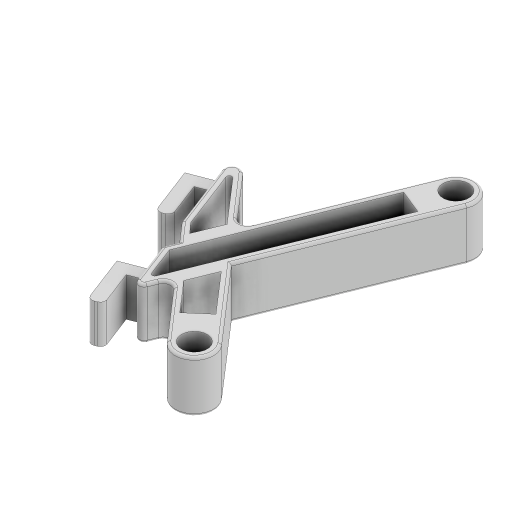
# Autodesk Inventor part: biellaa
Saved by Autodesk Inventor 2024 (Build 280153000, 153)
## iProperties
Created: 2024-04-18
Part Number: biellaa
Material: Generic
Document SubType Name: Modeling
Designer: alexz
Density: 1 g/cm^3
Appearance: Default
Author: alexz
Autodesk Inventor part; units mm, degrees
ref_plane "YZ Plane" through (0, 0, 0) normal (1, 0, 0) x (0, 1, 0)
ref_plane "XZ Plane" through (0, 0, 0) normal (0, 1, 0) x (-1, 0, 0)
ref_plane "XY Plane" through (0, 0, 0) normal (0, 0, 1) x (1, 0, 0)
sketch "Sketch1" plane through (0, 0, 0) normal (0, 1, 0) x (-1, 0, 0)
  circle A0 centre (0, 0) radius 5
  circle A1 centre (-0.0142, -101.8) radius 5
  circle A2 centre (0, 0) radius 7.5
  circle A3 centre (-0.0142, -101.8) radius 7.5001
  line L0 (0, 0) -> (51.0043, -58.881)
  line L1 (0, 0) -> (77.9, 0) construction
  line L2 (-0.0142, -101.8) -> (34.5269, -15.8763)
  line L3 (-0.0142, -101.8) -> (92.5923, -101.8) construction
  line L4 (-5.6689, -4.9106) -> (59.105, -79.6876)
  line L5 (6.9923, -104.4756) -> (76.3963, -104.4756) construction
  line L6 (-5.9244, -97.1825) -> (72.4099, -97.1825) construction
  line L7 (5.6689, 4.9106) -> (43.2486, -38.4727)
  line L8 (5.6689, 4.9106) -> (63.0653, 4.9106) construction
  line L9 (-6.958, -98.9653) -> (30.5885, -5.5656)
  line L10 (-6.958, -98.9653) -> (93.7061, -98.9653) construction
  line L11 (5.6547, -106.7106) -> (42.1064, -106.7106) construction
  line L12 (6.9446, -104.5974) -> (38.4943, -26.115)
  line L13 (6.9446, -104.5974) -> (92.3193, -104.5974) construction
  line L14 (30.5885, -5.5656) -> (38.4943, -26.115)
  line L15 (43.2486, -38.4727) -> (59.105, -79.6876)
  line L16 (51.0043, -58.881) -> (51.1768, -59.0801)
  point P0 (19.2756, -33.7073)
  point P1 (30.3178, -46.4547)
  point P2 (36.6082, -30.8068)
  point P3 (30.5165, -5.5798)
  point P4 (25.566, -18.0593)
  dimension "d0" = 10
  dimension "d1" = 10
  dimension "d2" = 101.8
  dimension "d3" = 15
  dimension "d14" = 77.9
  dimension "d15" = 49.1
  dimension "d17" = 68.1
  dimension "d20" = 49.1
  dimension "d21" = 68.1
  dimension "d23" = 68.1
  dimension "d24" = 22.0177
  dimension "d25" = 44.1598
  constraints: 35 end point, 8 horizontal, 7 point on circle, 4 centre point, 4 equal length, 3 coincident, 2 collinear, 2 tangent, 1 midpoint, 1 parallel, 1 other
  measures "d0" diameter of A0
  measures "d1" diameter of A1
  measures "d2" distance of A1.centre point (0, 0)
  measures "d3" diameter of A2
  measures "d14" distance of L0.start L0.end
  measures "d15" angle of L0 L1
  measures "d17" angle of L3 L2
  measures "d20" angle of L7 L8
  measures "d21" angle of L10 L9
  measures "d23" angle of L13 L12
  measures "d24" distance of L9.end L12.end
  measures "d25" distance of L7.end L4.end
extrude "Extrusion1" add sketch "Sketch1" along normal blind 20 contours A2 | A2 L7 L9 L0 | L0 L9 L4 A2 | L9 L14 L12 L7 | L7 L2 L0 L9 | L0 L2 L4 L9 | L4 L2 A3 L9 | L7 L12 L0 L2 | L0 L12 L4 L2 | L4 L12 A3 L2 | A3
fillet "Fillet1" radius 3 1 edges at (-25.566, 10, -18.0593)
sketch "Sketch12" plane through (6.958, 0, -98.9653) normal (0.9278363, 0, 0.3729878) x (0.3729878, 0, -0.9278363)
  line L0 (7.5402, 0) -> (0, 0) projected
  line L1 (7.5402, 0) -> (-7.4598, 0)
  line L2 (-7.4598, 0) -> (-7.4598, 5)
  line L3 (-7.4598, 5) -> (7.5402, 5)
  line L4 (7.5402, 5) -> (7.5402, 0)
  line L5 (-70.3336, 20) -> (0, 20) projected
  line L6 (-7.4598, 20) -> (7.5402, 20)
  line L7 (7.5402, 20) -> (7.5402, 15)
  line L8 (7.5402, 15) -> (-7.4598, 15)
  line L9 (-7.4598, 15) -> (-7.4598, 20)
  point P0 (-94.4189, 0)
  dimension "d74" = 15
  dimension "d75" = 5
  dimension "d76" = 15
  dimension "d77" = 5
  constraints: 16 end point, 4 parallel, 2 horizontal, 2 perpendicular, 2 point on line
  measures "d74" distance of L2.end L3.end
  measures "d75" distance of L1.end L2.end
  measures "d76" distance of L7.end L8.end
  measures "d77" distance of L6.end L7.end
extrude "Extrusion9" [suppressed]
sketch "Sketch13" plane through (-5.6689, 0, 4.9106) normal (-0.7558535, 0, 0.6547408) x (0.6547408, 0, 0.7558535)
  line L0 (7.5003, 0) -> (-7.4997, 0)
  line L1 (-7.4997, 0) -> (-7.4997, 5)
  line L2 (-7.4997, 5) -> (7.5003, 5)
  line L3 (7.5003, 5) -> (7.5003, 0)
  line L4 (0, 20) -> (-38.0983, 20) projected
  line L5 (-7.4997, 20) -> (7.5003, 20)
  line L6 (7.5003, 20) -> (7.5003, 15)
  line L7 (7.5003, 15) -> (-7.4997, 15)
  line L8 (-7.4997, 15) -> (-7.4997, 20)
  point P0 (0, 0)
  point P1 (0, 20)
  dimension "d80" = 15
  dimension "d81" = 5
  dimension "d82" = 15
  dimension "d83" = 5
  constraints: 16 end point, 4 parallel, 2 horizontal, 2 perpendicular, 2 point on line
  measures "d80" distance of L1.end L2.end
  measures "d81" distance of L0.end L1.end
  measures "d82" distance of L6.end L7.end
  measures "d83" distance of L5.end L6.end
extrude "Extrusion10" [suppressed]
sketch "Sketch16" plane through (0, 0, 0) normal (0, -1, 0) x (1, 0, 0)
  line L0 (-9.6603, -91.1392) -> (-0.3819, -87.4093)
  line L1 (-6.9446, -104.5974) -> (-38.4943, -26.115) projected
  line L2 (-0.3819, -87.4093) -> (-30.5374, -12.3953)
  line L3 (-30.5374, -12.3953) -> (-35.808, -26.0949)
  line L4 (-35.808, -26.0949) -> (-9.6603, -91.1392)
  line L5 (-19.2756, -33.7073) -> (-27.3992, -13.4992) projected
  line L6 (-38.4943, -26.115) -> (-30.5885, -5.5656) projected
  line L7 (3.8026, -91.1161) -> (-10.115, -96.7109) projected
  line L8 (-5.0595, -13.4775) -> (-12.6181, -6.9301)
  line L9 (-12.6181, -6.9301) -> (-22.6773, -18.5427)
  line L10 (-22.6773, -18.5427) -> (-18.4836, -28.9747)
  line L11 (-18.4836, -28.9747) -> (-5.0595, -13.4775)
  line L12 (-37.4002, -35.5394) -> (-40.9, -39.5796)
  line L13 (-40.9, -39.5796) -> (-51.4709, -67.0562)
  line L14 (-51.4709, -67.0562) -> (-33.2066, -45.9713)
  line L15 (-33.2066, -45.9713) -> (-37.4002, -35.5394)
  line L16 (-22.3481, -14.3445) -> (-5.6689, 4.9106) projected
  line L17 (5.6689, -4.9106) -> (-19.2756, -33.7073) projected
  line L18 (-22.3481, -14.3445) -> (-5.6689, 4.9106) projected
  line L19 (5.6689, -4.9106) -> (-19.2756, -33.7073) projected
  line L20 (-11.234, -1.514) -> (0.1038, -11.3351) projected
  point P0 (0, 0)
  point P1 (-28.4846, -51.0149)
  point P2 (-31.4986, -8.1805)
  point P3 (-36.6082, -30.8068)
  point P4 (-33.5357, -50.1696)
  point P5 (-47.711, -66.534)
  point P6 (-14.0085, -4.717)
  point P7 (-30.5885, -5.5656)
  point P8 (-30.3178, -46.4547)
  dimension "d87" = 5
  dimension "d88" = 2.5
  dimension "d89" = 2.5
  dimension "d90" = 2.5
  dimension "d95" = 2.5
  dimension "d96" = 2.5
  dimension "d97" = 5
  dimension "d98" = 5
  dimension "d99" = 5
  constraints: 24 end point, 10 parallel, 4 point on line, 3 perpendicular, 1 midpoint, 2 other
  measures "d87" distance between parallel lines of L7 L0
  measures "d88" distance between parallel lines of L5 L2
  measures "d89" distance between parallel lines of L4 L1
  measures "d95" distance between parallel lines of L17 L14
  measures "d96" distance from line of point (-14.009, -4.717) L12
  measures "d97" distance between parallel lines of L15 L4
  measures "d98" distance between parallel lines of L10 L2
  measures "d99" distance between parallel lines of L8 L20
extrude "Extrusion11" cut sketch "Sketch16" against normal through all contours L4 L3 L2 L0
fillet "Fillet10" radius 1 1 edges at (-30.5374, 10, -12.3953)
fillet "Fillet12" radius 2 1 edges at (-30.5885, 10, -5.5656)
extrude "Extrusion13" add sketch "Sketch1" along normal blind 20 contours L7 L15 L16 L0 L12 | L0 L16 L15 L4 L12
extrude "Extrusion14" cut sketch "Sketch16" against normal blind 20 contours L11 L10 L9 L8 | L15 L14 L13 L12
fillet "Fillet17" radius 1 1 edges at (-51.4709, 10, -67.0562)
fillet "Fillet18" radius 3 2 edges at (-59.105, 10, -79.6876) (-30.3178, 10, -46.4547)
fillet "Fillet19" radius 1 32 edges at (-30.773, 20, -49.175) (-40.7096, 20, -58.4514) (-51.6949, 20, -67.3412) (-48.0998, 20, -51.0822) (2.8303, 20, -108.7513) (-17.7146, 20, -77.8061) (-30.773, 0, -49.175) (-40.7096, 0, -58.4514) (-51.6949, 0, -67.3412) (-48.0998, 0, -51.0822) (2.8303, 0, -108.7513) (-17.7146, 0, -77.8061) (4.9106, 20, 5.6689) (-6.8033, 20, -19.3089) (-25.1108, 20, -15.3391) (-28.0456, 20, -11.8913) (-30.5626, 20, -9.0294) (-35.4543, 20, -18.2131) (-14.0085, 20, -4.717) (-6.1588, 20, -66.3363) (-39.9284, 20, -34.6397) (-37.5513, 20, -28.4609) (-37.5513, 0, -28.4609) (-39.9284, 0, -34.6397) (-6.1588, 0, -66.3363) (4.9106, 0, 5.6689) (-14.0085, 0, -4.717) (-25.1108, 0, -15.3391) (-28.0456, 0, -11.8913) (-30.5626, 0, -9.0294) (-35.4543, 0, -18.2131) (-6.8033, 0, -19.3089)
sketch "Sketch18" plane through (-32.4143, 1, -10.3112) normal (-0.9333118, 0, 0.3590671) x (0.3590671, 0, 0.9333118)
  line L0 (-3.51, 1.5) -> (-8.51, 1.5)
  line L1 (-8.51, 1.5) -> (-8.51, 16.5)
  line L2 (-8.51, 16.5) -> (-3.51, 16.5)
  line L3 (-3.51, 16.5) -> (-3.51, 1.5)
  line L4 (0, 18) -> (0, 0) projected
  line L5 (0, 0) -> (-16.933, 0)
  line L6 (-49.51, 1.5) -> (-54.51, 1.5)
  line L7 (-54.51, 1.5) -> (-54.51, 16.5)
  line L8 (-54.51, 16.5) -> (-49.51, 16.5)
  line L9 (-49.51, 16.5) -> (-49.51, 1.5)
  point P0 (21.2624, -1)
  point P1 (0, 9)
  point P2 (-3.51, 9)
  point P3 (-8.4665, 0)
  dimension "d123" = 5
  dimension "d124" = 15
  dimension "d125" = 5
  dimension "d126" = 46
  dimension "d129" = 3.51
  constraints: 18 end point, 4 parallel, 3 midpoint, 2 perpendicular, 1 horizontal, 1 horizontal alignment
  measures "d123" distance of L1.end L2.end
  measures "d124" distance of L0.end L1.end
  measures "d125" distance of L7.end L8.end
  measures "d126" distance between parallel lines of L7 L1
  measures "d129" distance between parallel lines of L3 L4
extrude "Extrusion15" add sketch "Sketch18" along normal blind 10
sketch "Sketch19" plane through (-33.6746, 2.5, -13.5871) normal (0.3590671, 0, 0.9333118) x (0.9333118, 0, -0.3590671)
  line L0 (-10, 15) -> (-10, 0) projected
  line L1 (-10, 0) -> (-5, 0)
  line L2 (-5, 0) -> (-5, 15)
  line L3 (-5, 15) -> (-10, 15)
  line L4 (-10, 15) -> (-10, 0)
  point P0 (26.5502, -2.5)
  dimension "d130" = 5
  dimension "d131" = 15
  constraints: 8 end point, 2 parallel, 1 horizontal, 1 perpendicular
  measures "d130" distance of L3.end L2.end
  measures "d131" distance of L2.end L1.end
sketch "Sketch20" plane through (-50.1917, 2.5, -56.5195) normal (0.3590671, 0, 0.9333118) x (0.9333118, 0, -0.3590671)
  line L0 (-10, 0) -> (-10, 15) projected
  line L1 (-10, 0) -> (-5, 0)
  line L2 (-5, 0) -> (-5, 15)
  line L3 (-5, 15) -> (-10, 15)
  line L4 (-10, 15) -> (-10, 0)
  point P0 (26.5502, -2.5)
  dimension "d132" = 5
  dimension "d133" = 15
  constraints: 8 end point, 2 parallel, 1 horizontal, 1 perpendicular
  measures "d132" distance of L3.end L2.end
  measures "d133" distance of L2.end L1.end
extrude "Extrusion16" add sketch "Sketch20" along normal blind 15
extrude "Extrusion17" add sketch "Sketch19" along normal blind 15
fillet "Fillet20" radius 2 4 edges at (-37.6217, 10, 4.0032) (-32.9551, 10, 2.2079) (-54.1388, 10, -38.9291) (-49.4722, 10, -40.7244)
body "Solid1"
